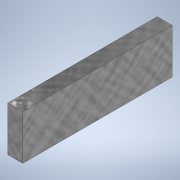
# Autodesk Inventor part: McCrea_obdlznicky_kos_walle_MIR2
Saved by Autodesk Inventor 2022 (Build 260153000, 153)
## iProperties
Created: 2022-02-08
Part Number: McCrea_obdlznicky_kos_walle_MIR2
Material: ABS Plastic
Document SubType Name: Modeling
Designer: Max
Density: 1.06 g/cm^3
Appearance: Honed - Dark Gray
Author: Max
Autodesk Inventor part; units mm, degrees
ref_plane "YZ Plane" through (0, 0, 0) normal (1, 0, 0) x (0, 1, 0)
ref_plane "XZ Plane" through (0, 0, 0) normal (0, 1, 0) x (-1, 0, 0)
ref_plane "XY Plane" through (0, 0, 0) normal (0, 0, 1) x (1, 0, 0)
sketch "Sketch1" plane through (0, 0, 0) normal (0, 0, 1) x (1, 0, 0)
  line L0 (-4.8066, 4.4492) -> (-4.3066, 4.4492)
  line L1 (-4.3066, 4.4492) -> (-4.3066, 2.9492)
  line L2 (-4.3066, 2.9492) -> (-4.8066, 2.9492)
  line L3 (-4.8066, 2.9492) -> (-4.8066, 4.4492)
  point P0 (0, 0)
  dimension "d0" = 1.5
  dimension "d1" = 0.5
  constraints: 8 end point, 2 parallel, 1 horizontal, 1 perpendicular
  measures "d0" distance of L0.end L1.end
  measures "d1" distance of L1.end L2.end
extrude "Extrusion1" add sketch "Sketch1" along normal blind 5
body "Solid1"
